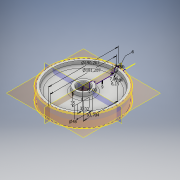
# Autodesk Inventor part: Колесо быстроходное
Saved by Autodesk Inventor 2018.3 (Build 223284000, 284)
## iProperties
Created: 2018-03-25
Part Number: Колесо быстроходное
Material: Типовые
Document SubType Name: Modeling
Designer: kriku
Density: 1 g/cm^3
Appearance: По умолчанию
Mass: 360.687 g
Surface Area: 862.831 cm^2
Volume: 360.687 cm^3
Author: kriku
Autodesk Inventor part; units mm, degrees
sketch "Эскиз1" plane through (0, 0, 0) normal (1, 0, 0) x (0, 1, 0)
  line L0 (0, 17.5) -> (0, -17.5)
  line L1 (16, 17.5) -> (16, -17.5)
  line L2 (90.6035, -17.5) -> (90.6035, 17.5)
  line L3 (93.7035, 17.5) -> (93.7035, -17.5)
  line L4 (95.1035, 16.3) -> (95.1035, -16.3)
  line L5 (90.6035, 17.5) -> (84.4535, 17.5)
  line L6 (84.4535, 17.5) -> (84.4535, 4.5)
  line L7 (77.5489, 4.5) -> (30.9046, 4.5)
  line L8 (24, 4.5) -> (24, 17.5)
  line L9 (24, 17.5) -> (16, 17.5)
  line L10 (90.6035, -17.5) -> (84.4535, -17.5)
  line L11 (84.4535, -17.5) -> (84.4535, -4.5)
  line L12 (77.5489, -4.5) -> (30.9046, -4.5)
  line L13 (24, -4.5) -> (24, -17.5)
  line L14 (24, -17.5) -> (16, -17.5)
  line L15 (114.0861, 0) -> (-18.3135, 0)
  line L16 (93.9035, 17.5) -> (90.6035, 17.5)
  line L17 (93.9035, -17.5) -> (90.6035, -17.5)
  line L18 (24, -17.5) -> (24.9493, -9.7688)
  line L19 (84.4535, -17.5) -> (83.5042, -9.7688)
  line L20 (84.4535, 17.5) -> (83.5042, 9.7688)
  line L21 (24, 17.5) -> (24.9493, 9.7688)
  arc A0 (83.5042, -9.7688) -> (77.5489, -4.5) centre (77.5489, -10.5) ccw
  arc A1 (30.9046, -4.5) -> (24.9493, -9.7688) centre (30.9046, -10.5) ccw
  arc A2 (24.9493, 9.7688) -> (30.9046, 4.5) centre (30.9046, 10.5) ccw
  arc A3 (77.5489, 4.5) -> (83.5042, 9.7688) centre (77.5489, 10.5) ccw
  line L22 (95.1035, 16.3) -> (93.9035, 17.5)
  line L23 (95.1035, -16.3) -> (93.9035, -17.5)
  line L24 (-44.7934, 0) -> (140.566, 0) projected
  point P0 (0, 0)
  dimension "d0" = 35
  dimension "d1" = 32
  dimension "d3" = 35
  dimension "d4" = 9
  dimension "d5" = 181.207
  dimension "d6" = 93.7035
  dimension "d7" = 190.207
  dimension "d9" = 6.15
  dimension "d10" = 48
  dimension "d11" = 7
  dimension "d12" = 7
  dimension "d13" = 7
  dimension "d14" = 6
  dimension "d15" = 6
  dimension "d16" = 135
  dimension "d17" = 1.2
  dimension "d18" = 135
  dimension "d19" = 1.2
  constraints: 48 end point, 11 point on line, 8 point on circle, 8 tangent, 7 perpendicular, 4 centre point, 4 parallel, 4 vertical, 2 equal radius, 2 horizontal, 2 symmetric about line, 1 midpoint, 2 other
  measures "d0" distance of L0.start L0.end
  measures "d1" diameter of L1 L0
  measures "d3" distance of L1.start L1.end
  measures "d4" distance between parallel lines of L12 L7
  measures "d5" diameter of L2 L0
  measures "d6" distance between parallel lines of L0 L3
  measures "d7" diameter of L4 L0
  measures "d9" distance from line of L10.end L2
  measures "d10" diameter of L13 L0
  measures "d11" angle of L11 L19
  measures "d12" angle of L20 L6
  measures "d13" angle of L13 L18
  measures "d14" radius of A0
  measures "d15" radius of A1
  measures "d16" angle of L4 L22
  measures "d17" horizontal distance of L16.start L4.start
  measures "d18" angle of L4 L23
  measures "d19" horizontal distance of L4.end L17.start
revolve "Вращение1" add sketch "Эскиз1" angle 360 about axis through (0, 0, 17.5) along (0, 0, -1) contours L9 L21 A2 L7 A3 L20 L5 L2 L15 L1 | L15 L2 L10 L19 A0 L12 A1 L18 L14 L1
surface revolve "ВращПврх1" sketch "Эскиз1" angle 360 about axis through (0, 0, 17.5) along (0, 0, -1) shown yes curves L16 L22 L4 L23 L17
chamfer "Фаска1" distance 1.6 angle 45 2 edges at (0, -16, 17.5) (0, -16, -17.5)
body "SRF1"
